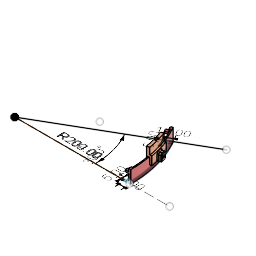
telescope complet (Autodesk Fusion 360 archive; units mm, degrees)
design "curseur_3"
Autodesk Fusion 360 part; units mm, degrees
(part 1 of 2)
sketch "Esquisse1" plane through (0, 0, 0) normal (0, 0, 1) x (1, 0, 0) in component "plateau bas"
  arc A0 (200, 0) -> (141.4214, 141.4214) centre (0, 0) ccw
  line L0 (0, 0) -> (200, 0) construction
  line L1 (0, 0) -> (141.4214, 141.4214) construction
  line L2 (0, 0) -> (141.4214, 141.4214)
  line L3 (0, 0) -> (200, 0)
  dimension "d1" = 200
  dimension "d2" = 45
  constraint coincident A0.centre L0.start
  measures "d1" radius of A0
  measures "d2" angle of L0 L1
extrude "Extrusion1" add sketch "Esquisse1" along normal blind 19 makes body 1 in component "plateau bas"
sketch "Esquisse1 (2)" plane through (0, 0, 0) normal (0, 0, 1) x (1, 0, 0) in component "plateau haut"
  line L0 (0, 0) -> (200, 0)
  arc A0 (200, 0) -> (141.4214, 141.4214) centre (0, 0) ccw
  line L1 (0, 0) -> (141.4214, 141.4214)
  point P0 (141.4214, 141.4214)
  constraint coincident L0.start A0.centre
  constraint horizontal L0
  constraint coincident P0 A0.end
extrude "Extrusion2" add sketch "Esquisse1 (2)" along normal blind 9 separate body makes body 2 in component "plateau haut"
sketch "Esquisse1 (3)" plane through (0, 0, 0) normal (0, 0, 1) x (1, 0, 0) in component "guide"
  line L0 (0, 0) -> (200, 0) construction
  line L1 (204, 0) -> (194, 0)
  line L2 (194, 5) -> (203.9387, 5)
  line L3 (194, 5) -> (194, 0)
  line L4 (0, 0) -> (235.9451, 136.223)
  line L5 (0, 0) -> (272.446, 0) construction
  arc A0 (200, 0) -> (173.2051, 100) centre (0, 0) ccw
  arc A1 (202, 0) -> (174.9371, 101) centre (0, 0) ccw
  arc A2 (204, 0) -> (176.6692, 102) centre (0, 0) ccw
  line L6 (176.6692, 102) -> (168.0089, 97)
  line L7 (168.0089, 97) -> (170.5089, 92.6699)
  line L8 (170.5089, 92.6699) -> (179.1161, 97.6392)
  arc A3 (187.7863, 74.4331) -> (187.1312, 81.2275) centre (81.8319, 67.6458) ccw
  dimension "d1_1" = 200
  dimension "d3_1" = 202
  dimension "d4_1" = 204
  dimension "d7" = 10
  dimension "d8" = 5
  dimension "d20" = 30
  dimension "d22" = 10
  dimension "d23" = 5
  constraint coincident L0.start L4.start
  constraint coincident L0 L1.end
  constraint parallel L0 L1
  constraint coincident L2.end A2
  constraint parallel L0 L2
  constraint perpendicular L0 L3
  constraint horizontal L5
  constraint coincident L4 A0.end
  constraint coincident L4 A1.end
  constraint coincident L4 A2.end
  constraint coincident L4 L6.end
  constraint perpendicular L6 L7
  constraint coincident A2 L8.end
  constraint perpendicular L7 L8
  constraint coincident A2 A3.end
  constraint coincident A1 A3.start
  measures "d1_1" radius of A0
  measures "d3_1" radius of A1
  measures "d4_1" radius of A2
  measures "d7" distance of L1.start L1.end
  measures "d8" distance of L1.end L2.start
  measures "d20" angle of L4 L5
  measures "d22" distance of A2.end L6.end
  measures "d23" distance of L6.end L7.end
extrude "Extrusion1'" add sketch "Esquisse1 (3)" along normal blind 10 separate body contours L1 L2 A0 A1 | L2 A0 A1 L8 | L4 A0 A1 L6 L8 makes body 3 in component "guide"
extrude "Extrusion2'" add sketch "Esquisse1 (3)" along normal blind 22 contours L1 L2 A1 A2 | L1 L2 A0 A1 | L2 A1 A2 A3 | A1 A2 L8 A3 | L4 A1 A2 L6 L8 | L4 A0 A1 L6 L8 bodies 3 in component "guide"
extrude "Extrusion3" add sketch "Esquisse1 (3)" along normal blind 17 and the other way blind -14 contours L1 L2 A0 A1 | L1 L2 L3 A0 | L4 A0 L6 L7 L8 | L4 A0 A1 L6 L8 bodies 3 in component "guide"
sketch "Esquisse1 (4)" plane through (0, 0, 0) normal (0, 0, 1) x (1, 0, 0) in component "curseur"
  line L0 (0, 0) -> (183.0742, 85.3689)
  arc A0 (183.0742, 85.3689) -> (165.4687, 115.8624) centre (0, 0) ccw
  line L1 (0, 0) -> (165.4687, 115.8624)
  arc A1 (181.2616, 84.5237) -> (163.8304, 114.7153) centre (0, 0) ccw
  line L2 (0, 0) -> (188.8449, 109.0297) construction
  line L3 (165.4687, 115.8624) -> (170.3836, 119.3039)
  line L4 (183.0742, 85.3689) -> (188.512, 87.9046)
  arc A2 (188.512, 87.9046) -> (170.3836, 119.3039) centre (0, 0) ccw
  line L5 (20, 0) -> (2.5, 0)
  arc A3 (185.7025, 86.5945) -> (167.8443, 117.5258) centre (0, 0) ccw
  line L6 (177.5812, 108.3001) -> (182.7774, 111.3001)
  line L7 (182.7774, 111.3001) -> (187.7774, 102.6398)
  line L8 (187.7774, 102.6398) -> (182.5812, 99.6398)
  line L9 (173.2051, 100) -> (178.7453, 100.1704)
  line L10 (173.2051, 100) -> (176.1228, 104.7128)
  dimension "d24_1" = 10
  dimension "d33" = 5
  dimension "d38" = 208
  dimension "d47" = 25
  dimension "d56" = 200
  dimension "d57" = 202
  dimension "d66" = 2.9
  dimension "d67" = 10
  dimension "d68" = 6
  constraint coincident L0 A1.start
  constraint coincident L1 A1.end
  constraint parallel L1 L3
  constraint parallel L0 L4
  constraint coincident L0.start A0.centre
  constraint coincident L0.start L2
  constraint coincident L0.start L1
  constraint coincident L0 A0.centre
  constraint coincident L4 A3.start
  constraint coincident L3 A3.end
  constraint coincident A2 L6.start
  constraint coincident A2 L8.end
  constraint perpendicular L7 L8
  constraint perpendicular L6 L7
  constraint perpendicular L2 L7
  constraint symmetric L2 L6 L8
  constraint midpoint A1 L9.start
  constraint coincident A3 L9.end
  constraint symmetric L2 L9.start L10.start
  constraint symmetric L2 L9.end L10.end
  measures "d24_1" angle of L0 L1
  measures "d33" angle of L0 L2
  measures "d38" radius of A2
  measures "d47" angle of L0 L5
  measures "d56" radius of A1
  measures "d57" radius of A0
  measures "d66" distance of A0 A3
  measures "d67" distance of L6.end L7.end
  measures "d68" distance of L7.end L8.end
extrude "Extrusion4" add sketch "Esquisse1 (4)" along normal blind 22 and the other way blind -10 separate body contours L0 A0 A1 L9 | A0 L1 A1 L10 | A0 L9 L10 | L3 L4 A2 A3 makes body 4 at (181.3843, 88.9029, 14) makes body 5 at (172.665, 115.9775, 18) in component "curseur"
extrude "Extrusion8" add sketch "Esquisse1 (4)" along normal blind 25 and the other way blind -22 contours L0 A0 A1 L9 | A0 L1 A1 L10 | A0 L4 A3 L9 | A0 L9 L10 | A0 L3 A3 L10 | A0 A3 L9 L10 | L3 L4 A2 A3 bodies 4 5 in component "curseur"
extrude "Extrusion5" add sketch "Esquisse1 (4)" along normal blind 37 and the other way blind -25 contours L0 A0 A1 L9 | A0 L1 A1 L10 | A0 L4 A3 L9 | A0 L9 L10 | A0 L3 A3 L10 | A0 A3 L9 L10 bodies 4 in component "curseur"
extrude "Extrusion9" add sketch "Esquisse1 (4)" along normal blind 40 and the other way blind -32 contours A0 L9 L10 | A0 A3 L9 L10 bodies 4 in component "curseur"
extrude "Extrusion10" add sketch "Esquisse1 (4)" along normal blind 22 and the other way blind -10 contours A2 L6 L7 L8 bodies 4 in component "curseur"
sketch "Esquisse2" plane through (185.2774, 106.9699, 0) normal (0.866025, 0.5, 0) x (-0.5, 0.866025, 0) in component "curseur"
  line L0 (-5, 10) -> (5, 10)
  line L1 (5, 10) -> (5, 22)
  line L2 (5, 22) -> (-5, 22)
  line L3 (-5, 22) -> (-5, 10)
  circle A0 centre (0, 16) radius 2.4
  dimension "d73" = 4.8
  measures "d73" diameter of A0
extrude "Extrusion11" cut sketch "Esquisse2" against normal blind 18 contours A0 bodies 4 in component "curseur"
fillet "Congé1" radius 2.5 2 edges at (180.1793, 109.8001, 22) (185.1793, 101.1398, 22) on bodies 4 in component "curseur"
fillet "Congé2" radius 1.5 5 edges at (182.5812, 99.6398, 14.75) (182.2292, 100.2821, 21.2678) (180.1333, 104, 22) (177.9615, 107.6741, 21.2678) (177.5812, 108.3001, 14.75) on bodies 4 in component "curseur"
fillet "Congé3" radius 1 5 edges at (187.7774, 102.6398, 14.75) (187.4113, 103.274, 21.2678) (185.2774, 106.9699, 22) (183.1435, 110.6659, 21.2678) (182.7774, 111.3001, 14.75) on bodies 4 in component "curseur"
component "plateau bas" placed x (1, 0, 0) y (0, 1, 0) z (0, 0, 1) at (0, 0, 0)
component "plateau haut" placed x (1, 0, 0) y (0, 1, 0) z (0, 0, 1) at (0, 0, 33)
component "guide" placed x (1, 0, 0) y (0, 1, 0) z (0, 0, 1) at (0, 0, 5)
component "curseur" placed x (0.965926, -0.258819, 0) y (0.258819, 0.965926, 0) z (0, 0, 1) at (0, 0, 5)
named bodies: "guide"

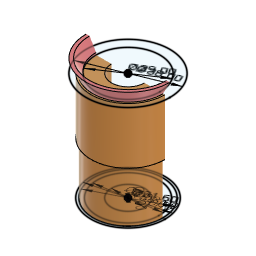
design "oculaire_20mm"
Autodesk Fusion 360 part; units mm, degrees
sketch "Esquisse1" plane through (0, 0, 0) normal (0, 0, 1) x (1, 0, 0)
  circle A0 centre (0, 0) radius 15.8
  circle A1 centre (0, 0) radius 16.8
  circle A2 centre (0, 0) radius 14
  circle A3 centre (0, 0) radius 7.5
  circle A4 centre (0, 0) radius 1
  dimension "d1" = 31.6
  dimension "d2" = 33.6
  dimension "d3" = 28
  dimension "d10" = 15
  dimension "d11" = 2
  constraint coincident A0.centre A1.centre
  constraint concentric A3 A4
  measures "d1" diameter of A0
  measures "d2" diameter of A1
  measures "d3" diameter of A2
  measures "d10" diameter of A3
  measures "d11" diameter of A4
extrude "Extrusion1" add sketch "Esquisse1" along normal blind 23.5 contours A0 makes body 1
extrude "Extrusion2" add sketch "Esquisse1" along normal blind 49 and the other way blind -23.5 contours A0 | A1 | A2 bodies 1
extrude "Extrusion4" add sketch "Esquisse1" along normal blind 40 and the other way blind -36 separate body contours A3 | A4 makes body 2
chamfer "Chanfrein1" distance 7 distance2 2 1 edges at (-6.9925, -2.7121, 40) measured on face at (1.9158, 2.8099, 40) on bodies 2
chamfer "Chanfrein2" distance 1.5 distance2 7 1 edges at (-6.9925, -2.7121, 36) measured on face at (7.4627, -0.7468, 36.6667) on bodies 2
extrude "Extrusion3" add sketch "Esquisse1" along normal blind 43 and the other way blind -23 separate body contours A4 makes body 3
sketch "Esquisse1 (2)" plane through (0, 0, 0) normal (0, 0, 1) x (1, 0, 0) in component "cahoutchouc"
  circle A0 centre (0, 0) radius 14.5
  circle A1 centre (0, 0) radius 19
  dimension "d24" = 29
  dimension "d25" = 38
  constraint coincident A0.centre A1.centre
  measures "d24" diameter of A0
  measures "d25" diameter of A1
extrude "Extrusion1'" add sketch "Esquisse1 (2)" along normal blind 6 separate body makes body 4 in component "cahoutchouc"
chamfer "Chanfrein1'" distance 3 distance2 5 1 edges at (-13.5187, 5.2434, 6) measured on face at (17.3753, -1.6643, 6) on bodies 4 in component "cahoutchouc"
chamfer "Chanfrein2'" distance 6 distance2 3 1 edges at (-17.7142, -6.8707, 0) measured on face at (18.9764, -0.9471, 4) on bodies 4 in component "cahoutchouc"
component "cahoutchouc" placed x (1, 0, 0) y (0, 1, 0) z (0, 0, 1) at (0, 0, 49)

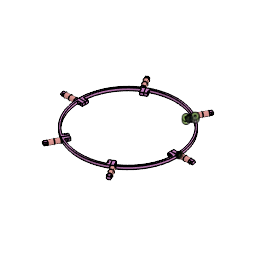
design "table a rouleau3"
Autodesk Fusion 360 part; units mm, degrees
sketch "Esquisse1" plane through (0, 0, 0) normal (0, 0, 1) x (1, 0, 0)
  line L0 (130.5, 0) -> (150, 0) construction
  arc A0 (46, 0) -> (45.9562, 2.0065) centre (0, 0) ccw
  arc A1 (47.9583, 2) -> (47.9543, 2.0937) centre (0, 0) ccw
  line L1 (130.5, 0) -> (150, 0)
  line L2 (80.1544, 120.8316) -> (72.8889, 108.2472)
  line L3 (144.7204, 9) -> (130.1893, 9)
  arc A2 (150, 0) -> (75, 129.9038) centre (0, 0) ccw
  arc A3 (144.7204, 9) -> (80.1544, 120.8316) centre (0, 0) ccw
  line L4 (186.382, -4.6913) -> (189.3792, -4.5604)
  line L5 (147.0059, 71.8492) -> (150.8185, -15.4747) construction
  line L6 (0, 0) -> (371.6459, 16.2264) construction
  line L7 (185.2639, 20.9177) -> (188.2563, 21.1586)
  line L8 (185.2639, 20.9177) -> (186.382, -4.6913)
  line L9 (188.2563, 21.1586) -> (189.3792, -4.5604)
  line L10 (65.25, 113.0163) -> (75, 129.9038)
  arc A4 (130.5, 0) -> (130.1893, 9) centre (0, 0) ccw
  arc A5 (72.8889, 108.2472) -> (65.25, 113.0163) centre (0, 0) ccw
  dimension "d2" = 150
  dimension "d6" = 46
  dimension "d7" = 48
  dimension "d13" = 145
  dimension "d49" = 2.5
  dimension "d64" = 3
  dimension "d65" = 186
  dimension "d70" = 9
  dimension "d71" = 9
  dimension "d80" = 261
  constraint horizontal L0
  constraint coincident A0.centre A1.centre
  constraint perpendicular L5 L6
  constraint tangent A2 L5
  constraint perpendicular L4 L8
  constraint perpendicular L4 L9
  constraint perpendicular L6 L8
  constraint midpoint L6 L8
  constraint coincident L6 A1.end
  constraint coincident L6 A0.end
  constraint concentric A1 A4
  constraint concentric A4 A5
  measures "d2" distance of A0.centre A2.end
  measures "d6" radius of A0
  measures "d7" radius of A1
  measures "d13" radius of A3
  measures "d49" angle of L1 L6
  measures "d64" distance of L8 L9
  measures "d65" distance of A0.centre L8
  measures "d70" distance of L2 L10
  measures "d71" distance of L1 L3
  measures "d80" diameter of A4
extrude "Extrusion1" add sketch "Esquisse1" along normal blind 8 contours L1 L2 L3 A2 A3 L10 A4 A5 makes body 1
sketch "Esquisse3" plane through (0, 0, 0) normal (-0.866025, 0.5, 0) x (-0.5, -0.866025, 0)
  line L0 (-144.5026, 0) -> (-129.5026, 0)
  line L1 (-129.5026, 0) -> (-129.5026, 8)
  line L2 (-129.5026, 8) -> (-144.5026, 8)
  line L3 (-144.5026, 8) -> (-144.5026, 0)
  circle A0 centre (-137.0026, 4) radius 2.2
  line L4 (-133.2026, 6.1939) -> (-137.0026, 8.3879)
  line L5 (-137.0026, 8.3879) -> (-140.8026, 6.1939)
  line L6 (-140.8026, 6.1939) -> (-140.8026, 1.8061)
  line L7 (-140.8026, 1.8061) -> (-137.0026, -0.3879)
  line L8 (-137.0026, -0.3879) -> (-133.2026, 1.8061)
  line L9 (-133.2026, 1.8061) -> (-133.2026, 6.1939)
  line L10 (-129.5026, 0) -> (-150, 0)
  line L11 (-150, 8) -> (-129.5026, 8)
  line L12 (-150, 0) -> (-150, 8)
  line L13 (-150, 0) -> (-130.5, 0)
  line L14 (-130.5, 8) -> (-150, 8)
  line L15 (-150, 8) -> (-150, 0)
  line L16 (-130.5, 0) -> (-130.5, 8)
  point P0 (-137.0026, 4)
  dimension "d32" = 4.4
  dimension "d33" = 7.5
  dimension "d34" = 4
  dimension "d35" = 3.8
  constraint coincident P0 A0.centre
  measures "d32" diameter of A0
  measures "d33" distance of L1 P0
  measures "d34" distance of L0 P0
  measures "d35" distance of P0 L9
extrude "Extrusion4" cut sketch "Esquisse3" along normal mid plane 30 contours A0 bodies 1
extrude "Extrusion5" cut sketch "Esquisse3" along normal blind -7 and the other way blind 15 contours L0 L2 L4 L5 L6 L7 L8 L9 L10 L11 L13 L14 bodies 1
pattern_circular "Réseau C1" count 2 over 60 about axis through (0, 0, 8) along (0, 0, -1) of "Extrusion4"
ref_plane "Plan de construction2" through (148.9122, 28.1873, 0) normal (0.999048, 0.043619, 0) x (0.043619, -0.999048, 0)
sketch "Esquisse2" plane through (149.8572, 6.5429, 0) normal (0.999048, 0.043619, 0) x (-0.043619, 0.999048, 0)
  line L0 (0, 0) -> (6, 0)
  line L1 (6, 0) -> (6, 8)
  line L2 (6, 8) -> (0, 8)
  line L3 (0, 8) -> (0, 0)
  circle A0 centre (0, 4) radius 5.5
  circle A1 centre (0, 4) radius 6.5
  line L4 (-5.1235, 0) -> (5.1235, 0)
  line L5 (-5.1235, 8) -> (5.1235, 8)
  dimension "d25" = 11
  dimension "d26" = 13
  dimension "d27" = 4
  constraint midpoint L3 A0.centre
  constraint concentric A0 A1
  constraint coincident A1 L4.start
  constraint coincident A1 L4.end
  constraint coincident L0 L4.end
  constraint parallel L0 L4
  constraint coincident A1 L5.start
  constraint coincident A1 L5.end
  constraint parallel L2 L5
  measures "d25" diameter of A0
  measures "d26" diameter of A1
  measures "d27" distance of A0.centre L5
extrude "Extrusion2" add sketch "Esquisse2" along normal blind 42 contours L0 L2 L3 A0 L4 L5 | L3 A0 L4 L5 bodies 1
extrude "Extrusion3" add sketch "Esquisse2" along normal blind 3 contours L0 L1 L2 A0 A1 L4 L5 | A0 A1 L4 L5 | L1 A1 bodies 1
extrude "Extrusion7" cut sketch "Esquisse1" along normal blind 5.5 and the other way blind -2.5 contours L4 L7 L8 L9 bodies 1
sketch "Esquisse1 (2)" plane through (0, 0, 0) normal (0, 0, 1) x (1, 0, 0) in component "rouleau"
  circle A0 centre (0, 0) radius 6
  circle A1 centre (0, 0) radius 7
  dimension "d55" = 12
  dimension "d56" = 14
  constraint coincident A0.centre A1.centre
  constraint concentric A0 A1
  measures "d55" diameter of A0
  measures "d56" diameter of A1
extrude "Extrusion1'" add sketch "Esquisse1 (2)" along normal blind 30 separate body makes body 2 in component "rouleau"
extrude "Extrusion2'" cut 1 faces at (6.6406, -0.3478, 0) along direction (0, 0, -1) blind -15.2 and the other way blind 14.8 on bodies 2 bodies 2 makes body 3 at (6.9652, -0.697, 25.0667) in component "rouleau"
pattern_circular "Réseau C2" count 6 over 360 about axis through (0, 0, 0) along (0, 0, 1) of bodies 1 makes body 4 at (56.2488, 139.0542, 5.3333) makes body 5 at (-92.3001, 118.24, 5.3333) makes body 6 at (-149.3736, -13.6942, 2.6667) makes body 7 at (-62.8273, -136.2084, 2.6667) makes body 8 at (92.3001, -118.24, 5.3333)
component_pattern "component pattern"
component "rouleau" placed x (0, 0, -1) y (0.043619, -0.999048, 0) z (-0.999048, -0.043619, 0) at (182.8258, 7.9823, 4)
component "rouleau" placed x (0, 0, -1) y (0.887011, -0.461749, 0) z (-0.461749, -0.887011, 0) at (84.5, 162.323, 4)
component "rouleau" placed x (0, 0, -1) y (0.843391, 0.5373, 0) z (0.5373, -0.843391, 0) at (-98.3258, 154.3406, 4)
component "rouleau" placed x (0, 0, -1) y (-0.043619, 0.999048, 0) z (0.999048, 0.043619, 0) at (-182.8258, -7.9823, 4)
component "rouleau" placed x (0, 0, -1) y (-0.887011, 0.461749, 0) z (0.461749, 0.887011, 0) at (-84.5, -162.323, 4)
component "rouleau" placed x (0, 0, -1) y (-0.843391, -0.5373, 0) z (-0.5373, 0.843391, 0) at (98.3258, -154.3406, 4)

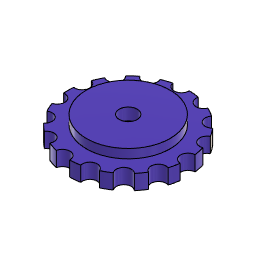
design "molette_ecrou_6"
Autodesk Fusion 360 part; units mm, degrees
sketch "Esquisse2" plane through (0, 0, 0) normal (0, 0, 1) x (1, 0, 0)
  circle A0 centre (0, 0) radius 14
  circle A1 centre (0, 0) radius 20
  circle A2 centre (20, 0) radius 2.5
  line L0 (0.202, 5.77) -> (-4.8959, 3.06)
  line L1 (-4.8959, 3.06) -> (-5.098, -2.71)
  line L2 (-5.098, -2.71) -> (-0.202, -5.77)
  line L3 (-0.202, -5.77) -> (4.8959, -3.06)
  line L4 (4.8959, -3.06) -> (5.098, 2.71)
  line L5 (5.098, 2.71) -> (0.202, 5.77)
  circle A3 centre (0, 0) radius 3
  dimension "d51_1" = 40
  dimension "d52_1" = 28
  dimension "d53_1" = 5
  dimension "d2_2" = 5
  dimension "d7_2" = 6
  constraint coincident A0.centre A1.centre
  measures "d51_1" diameter of A1
  measures "d52_1" diameter of A0
  measures "d53_1" diameter of A2
  measures "d2_2" distance of A0.centre L5
  measures "d7_2" diameter of A3
extrude "Extrusion1" add sketch "Esquisse2" along normal blind 5 contours A0 | A1 A2 | A1 A2 | L0 L1 L2 L3 L4 L5 picked at (19.214, -0.5707) picked at (17.0514, 3.8379)
extrude "Extrusion2" add sketch "Esquisse2" along normal blind 8 contours A0 | L0 L1 L2 L3 L4 L5
extrude "Extrusion3" cut sketch "Esquisse2" along normal blind 4 contours L0 L1 L2 L3 L4 L5
extrude "Extrusion6" cut sketch "Esquisse2" along normal blind 5 contours A1 A2 picked at (19.214, -0.5707)
pattern_circular "Réseau C1" count 15 over 360 about axis through (0, 0, 0) along (0, 0, 1) of "Extrusion6"

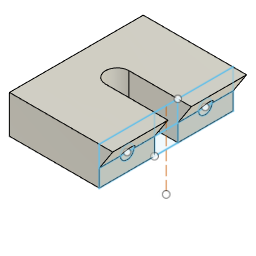
design "cale"
Autodesk Fusion 360 part; units mm, degrees
sketch "Esquisse1" plane through (-35, -25, 52.8) normal (-1, 0, 0) x (0, -1, 0)
  line L0 (14.952, -3.6934) -> (-14.848, -3.6934)
  line L1 (0.052, -3.6934) -> (0.052, -20.8144) construction
  circle A0 centre (8.7476, -8.3) radius 1.5
  circle A1 centre (-8.6437, -8.3) radius 1.5
  line L2 (-14.848, -12.1415) -> (14.952, -12.1415)
  line L3 (2.652, -3.6934) -> (2.652, -12.1415)
  line L4 (-2.548, -3.6934) -> (-2.548, -12.1415)
  line L5 (14.952, -8.3) -> (-14.848, -8.3)
  line L6 (14.952, -3.6934) -> (14.952, -12.1415)
  line L7 (-14.848, -3.6934) -> (-14.848, -12.1415)
  dimension "d166" = 3
  dimension "d167" = 2.6
  dimension "d194" = 14.9
  constraint vertical L1
  constraint symmetric L1 A0 A1
  constraint coincident L0 L3.start
  constraint perpendicular L0 L3
  constraint symmetric L1 L3.start L4.start
  constraint symmetric L1 L3.end L4.end
  constraint coincident L2 L4.end
  constraint perpendicular L2 L4
  constraint perpendicular L2 L6
  constraint symmetric L1 L0.start L0.end
  constraint symmetric L1 L2.end L2.start
  constraint coincident L0 L1.start
  constraint coincident L7 L5.end
  constraint coincident L6 L5.start
  measures "d166" diameter of A0
  measures "d167" distance of L1 L3
  measures "d194" distance of L1 L6
extrude "Extrusion1" add sketch "Esquisse1" along normal blind 20 and the other way blind 3 contours L0 A0 L3 L5 L6 | L0 L3 L4 L5 | L0 A1 L4 L5 L7
extrude "Extrusion3" add sketch "Esquisse1" along normal blind 20 contours A0 L2 L3 L5 L6 | L2 L3 L4 L5 | A1 L2 L4 L5 L7
chamfer "Chanfrein1" distance 4.6 distance2 3 3 edges at (-32, -37.5998, 44.5) (-32, -25.052, 44.5) (-32, -12.5041, 44.5) measured on face at (-32, -22.2647, 48.0585) measured on face at (-32, -22.2647, 48.0585) measured on face at (-32, -22.2647, 48.0585)
extrude "Extrusion4" cut sketch "Esquisse1" along normal blind 13.5 and the other way blind 3 contours L0 L3 L4 L5 | L2 L3 L4 L5
fillet "Congé1" radius 2.6 2 edges at (-48.5, -22.452, 44.8825) (-48.5, -27.652, 44.8825)

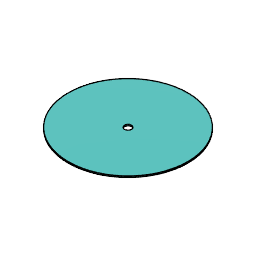
design "plaque"
Autodesk Fusion 360 part; units mm, degrees
sketch "Esquisse1" plane through (0, 0, 0) normal (0, 0, 1) x (1, 0, 0)
  circle A0 centre (0, 0) radius 70
  circle A1 centre (0, 0) radius 4.1
  dimension "d1" = 140
  dimension "d2" = 8.2
  constraint coincident A0.centre A1.centre
  constraint concentric A0 A1
  measures "d1" diameter of A0
  measures "d2" diameter of A1
extrude "Extrusion1" add sketch "Esquisse1" along normal blind 1.5
equation "d5 = 8bf455b0-8dd7-4d48-b475-9f234ed07525"

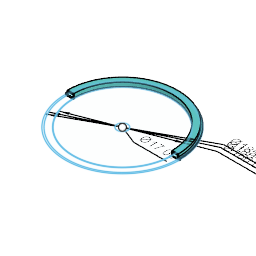
design "roulement3ext"
Autodesk Fusion 360 part; units mm, degrees
sketch "Esquisse3" plane through (0, 0, 0) normal (0, 0, 1) x (1, 0, 0)
  circle A0 centre (0, 0) radius 80
  circle A1 centre (0, 0) radius 90
  circle A2 centre (0, 0) radius 92.5
  circle A3 centre (0, 0) radius 8.5
  circle A4 centre (0, 0) radius 79.9
  dimension "d28" = 160
  dimension "d29" = 180
  dimension "d30" = 185
  dimension "d33" = 17
  constraint concentric A0 A1
  constraint concentric A1 A2
  measures "d28" diameter of A0
  measures "d29" diameter of A1
  measures "d30" diameter of A2
  measures "d33" diameter of A3
extrude "Extrusion1" add sketch "Esquisse3" along normal blind 2.5 and the other way blind -0.5 contours A1 | A2
extrude "Extrusion2" add sketch "Esquisse3" along normal blind 7 and the other way blind -0.5 contours A1
named bodies: "Corps1"

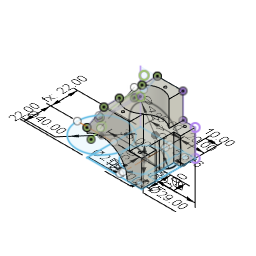
design "Bati"
Autodesk Fusion 360 part; units mm, degrees
sketch "Esquisse1" plane through (0, 0, 23) normal (0, 0, 1) x (-1, 0, 0)
  line L0 (-10, 3) -> (-10, 47)
  line L1 (-10, 47) -> (35, 47)
  line L2 (65, 25) -> (35, 25) construction
  circle A0 centre (10, 25) radius 14.5
  line L3 (10, 3.7685) -> (10, 45.0557) construction
  circle A1 centre (10, 42.5) radius 1
  line L4 (35, 3) -> (-10, 3)
  circle A2 centre (10, 7.5) radius 1
  circle A3 centre (45, 25) radius 20
  line L5 (35, 47) -> (35, 3)
  line L6 (0, 47) -> (0, 3)
  circle A4 centre (-5, 43.5) radius 1
  circle A5 centre (-5, 6.5) radius 1
  line L7 (-10, 15) -> (-4.3838, 15)
  line L8 (-4.3838, 15) -> (-4.3838, 35)
  line L9 (-4.3838, 35) -> (-10, 35)
  dimension "d71" = 29
  dimension "d72" = 20
  dimension "d75" = 17.5
  dimension "d85" = 40
  dimension "d93" = 35
  dimension "d94" = 22
  dimension "d95" = 22
  dimension "d96" = 25
  dimension "d115" = 10
  dimension "d120" = 2
  dimension "d121" = 2
  dimension "d140" = 18.5
  dimension "d141" = 5.6162
  dimension "d142" = 10
  constraint horizontal L1
  constraint coincident L2 A0.centre
  constraint coincident A0.centre L3
  constraint perpendicular L0 L4
  constraint symmetric L2 A1 A2
  constraint coincident L2 A3.centre
  constraint perpendicular L4 L5
  constraint coincident L1 L6.start
  constraint coincident L4 L6.end
  constraint perpendicular L4 L6
  constraint symmetric L2 A4 A5
  constraint coincident L0 L7.start
  constraint perpendicular L0 L7
  constraint perpendicular L7 L8
  constraint coincident L0 L9.end
  constraint perpendicular L0 L9
  constraint symmetric L2 L7 L9
  measures "d71" diameter of A0
  measures "d72" distance of L0 A0.centre
  measures "d75" distance of L2 A1.centre
  measures "d85" diameter of A3
  measures "d93" distance of A0.centre A3.centre
  measures "d94" distance of L1 L2
  measures "d95" distance of L2 L4
  measures "d96" distance of L3 L5
  measures "d115" distance of L0 L6
  measures "d120" diameter of A4
  measures "d121" diameter of A1
  measures "d140" distance of L2 A4.centre
  measures "d141" distance of L7.start L7.end
  measures "d142" distance of L2 L9
extrude "Extrusion1" add sketch "Esquisse1" along normal blind 43 contours L0 A0 L4 L6 L7 L8 | L1 A0 L4 A3 L5 L6 | L0 L1 A0 L6 L8 L9 | A0 L6 | A0 L6 L8 | A0 L8 | A3 L5 picked at (30.9179, 24.5677)
extrude "Extrusion4" cut sketch "Esquisse1" along normal blind 55 and the other way blind -26 contours A3 L5 picked at (30.9179, 24.5677)
extrude "Extrusion7" cut sketch "Esquisse1" along normal blind 50 and the other way blind -22 contours L0 A0 L4 L6 L7 L8 | L0 A0 L7 L8 L9 | L0 L1 A0 L6 L8 L9 | A0 L6 | A0 L6 L8 | A0 L8 | A4 | A5
sketch "Esquisse2" plane through (0, -3, 0) normal (0, 1, 0) x (-1, 0, 0)
  line L0 (35, 66) -> (0, 66)
  line L1 (-10, 23) -> (35, 23)
  circle A0 centre (23, 23) radius 21.35
  line L2 (-10, 23) -> (-10, 45)
  line L3 (35, 23) -> (35, 66)
  line L4 (21.0907, 66) -> (35, 44.5)
  line L5 (0, 66) -> (0, 45)
  line L6 (0, 45) -> (-10, 45)
  line L7 (-10, 45) -> (-10, 23)
  dimension "d104" = 42.7
  dimension "d105" = 33
  constraint coincident L1 A0.centre
  constraint coincident L0 L4.start
  constraint midpoint L3 L4.end
  measures "d104" diameter of A0
  measures "d105" distance of A0.centre L2
extrude "Extrusion5" cut sketch "Esquisse2" against normal blind 55 draft -0.45 contours L1 A0 L3 | L1 A0 L3
extrude "Extrusion8" cut sketch "Esquisse2" against normal blind 50 contours L0 L3 L4
sketch "Esquisse3" plane through (-44.9682, 0, 29.0918) normal (-0.839615, 0, 0.543183) x (0, -1, 0)
  line L0 (47, 18.3515) -> (47, 43.9584)
  line L1 (47, 43.9584) -> (34.3405, 43.9584)
  line L2 (15.6595, 43.9584) -> (3, 43.9584)
  line L3 (3, 43.9584) -> (3, 18.3515)
  line L4 (3, 18.3515) -> (47, 18.3515)
  ellipse E0 centre (25, -0.0586) end of major axis (25, -35.0376) minor radius 19 (38.9391, 23.7111) -> (11.0609, 23.7111) ccw
  line L5 (25, 49.3303) -> (25, -2) construction
  circle A0 centre (43.5, 30) radius 1.5
  circle A1 centre (6.5, 30) radius 1.5
  ellipse E1 centre (25, 64.3765) end of major axis (25, 37.682) minor radius 14.5 (15.6595, 43.9584) -> (34.3405, 43.9584) ccw
  line L6 (38.9391, 23.7111) -> (11.0609, 23.7111)
  line L7 (25, -15.9957) -> (25, 0.2997)
  line L8 (47, 18.3515) -> (47, 43.9584)
  line L9 (47, 43.9584) -> (34.3405, 43.9584)
  ellipse E2 centre (25, 64.3765) end of major axis (25, 37.682) minor radius 14.5 (15.6595, 43.9584) -> (34.3405, 43.9584) ccw
  line L10 (15.6595, 43.9584) -> (3, 43.9584)
  line L11 (3, 43.9584) -> (3, 18.3515)
  line L12 (3, 18.3515) -> (47, 18.3515)
  ellipse E3 centre (25, -0.0586) end of major axis (25, -36.8786) minor radius 20 (40.2742, 23.7111) -> (9.7258, 23.7111) ccw
  line L13 (40.2742, 23.7111) -> (9.7258, 23.7111)
  dimension "d112" = 3
  dimension "d139" = 18.5
  constraint perpendicular L4 L5
  constraint symmetric L5 A0 A1
  constraint coincident L5 L7.start
  measures "d112" diameter of A0
  measures "d139" distance of L5 A0.centre
extrude "Extrusion6" cut sketch "Esquisse3" against normal blind 12 contours A0 | A1
equation "d95 = d94"

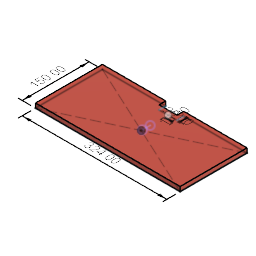
design "plaque avant"
Autodesk Fusion 360 part; units mm, degrees
sketch "Esquisse1" plane through (0, 0, 0) normal (0, 0, 1) x (1, 0, 0)
  line L0 (-162, 75) -> (-162, -75)
  line L1 (-162, -75) -> (162, -75)
  line L2 (162, -75) -> (162, 75)
  line L3 (162, 75) -> (-162, -75) construction
  line L4 (-162, 75) -> (162, -75) construction
  line L5 (20, 75) -> (20, 60)
  line L6 (20, 60) -> (0, 60)
  line L7 (0, 2.5) -> (0, 20)
  line L8 (-20, 75) -> (-20, 60)
  line L9 (-20, 60) -> (0, 60)
  line L10 (162, 75) -> (20, 75)
  line L11 (-20, 75) -> (-162, 75)
  dimension "d1" = 324
  dimension "d2" = 150
  dimension "d5" = 15
  dimension "d6" = 20
  constraint horizontal L10
  constraint perpendicular L0 L10
  constraint parallel L1 L10
  constraint parallel L0 L2
  constraint coincident L3 origin
  constraint coincident L4 origin
  constraint perpendicular L5 L10
  constraint perpendicular L5 L6
  constraint symmetric L5.start L7 L8.start
  constraint symmetric L5.end L7 L8.end
  constraint symmetric L6.end L7 L9.end
  constraint collinear L10 L11
  measures "d1" distance of L0.end L1.end
  measures "d2" distance of L0.start L0.end
  measures "d5" distance of L5.start L5.end
  measures "d6" distance of L5.end L6.end
extrude "Extrusion1" add sketch "Esquisse1" along normal blind 10

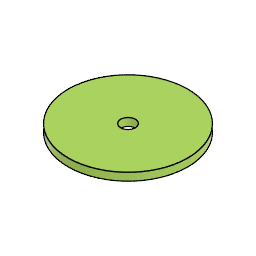
design "plaque de serrage"
Autodesk Fusion 360 part; units mm, degrees
sketch "Esquisse1" plane through (0, 0, 0) normal (0, 0, 1) x (1, 0, 0)
  circle A0 centre (0, 0) radius 69
  circle A1 centre (0, 0) radius 8.5
  dimension "d1" = 138
  dimension "d2" = 17
  constraint coincident A0.centre A1.centre
  constraint concentric A0 A1
  measures "d1" diameter of A0
  measures "d2" diameter of A1
extrude "Extrusion1" add sketch "Esquisse1" along normal blind 9

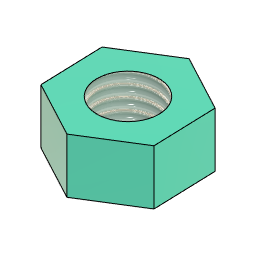
design "ecrou"
Autodesk Fusion 360 part; units mm, degrees
sketch "Esquisse1" plane through (0, 0, 0) normal (0, 0, 1) x (1, 0, 0)
  circle A0 centre (0, 0) radius 4
  line L0 (-0.2292, 6.9244) -> (-6.1113, 3.2637)
  line L1 (-6.1113, 3.2637) -> (-5.8821, -3.6607)
  line L2 (-5.8821, -3.6607) -> (0.2292, -6.9244)
  line L3 (0.2292, -6.9244) -> (6.1113, -3.2637)
  line L4 (6.1113, -3.2637) -> (5.8821, 3.6607)
  line L5 (5.8821, 3.6607) -> (-0.2292, 6.9244)
  dimension "d1" = 8
  dimension "d2" = 6
  constraint coincident A0.centre origin
  measures "d1" diameter of A0
  measures "d2" distance of A0.centre L5
extrude "Extrusion1" add sketch "Esquisse1" along normal blind 6
thread "Filetage1" "ISO Metric profile 8.0 M8x1.25 6H" major diameter 8.17 minor diameter 6.7795 pitch 1.25 angle 60 resizes the face on face at (3.995, -0.1994, 4)

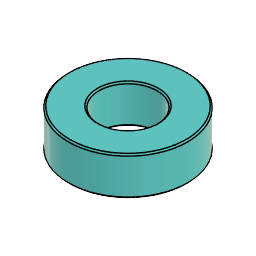
design "interieur_grand_pignon"
Autodesk Fusion 360 part; units mm, degrees
sketch "Esquisse1" plane through (0, 0, 0) normal (0, 0, 1) x (1, 0, 0)
  circle A0 centre (0, 0) radius 11
  circle A1 centre (0, 0) radius 4.1
  circle A2 centre (0, 0) radius 8.4
  dimension "d1" = 22
  dimension "d2" = 8.2
  dimension "d5" = 16.8
  constraint coincident A0.centre A1.centre
  constraint concentric A0 A1
  constraint concentric A1 A2
  measures "d1" diameter of A0
  measures "d2" diameter of A1
  measures "d5" diameter of A2
extrude "Extrusion1" add sketch "Esquisse1" along normal blind 5.4 contours A2
chamfer "Chanfrein1" distance 0.2 angle 45 4 edges at (-3.8225, 1.4826, 5.4) (-3.8225, 1.4826, 0) (-7.8315, -3.0376, 5.4) (-7.8315, -3.0376, 0)

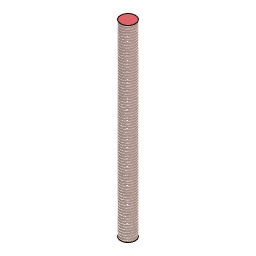
design "tige"
Autodesk Fusion 360 part; units mm, degrees
sketch "Esquisse1" plane through (0, 0, 0) normal (0, 0, 1) x (0, -1, 0)
  circle A0 centre (0, 0) radius 4
  dimension "d44" = 8
  constraint coincident A0.centre origin
  measures "d44" diameter of A0
extrude "Extrusion1" add sketch "Esquisse1" along normal blind 100
thread "Filetage1" "ISO Metric profile 8.0 M8x1.25 6g" major diameter 7.866 minor diameter 6.4455 pitch 1.25 angle 60 resizes the face on face at (-0.3983, -3.9801, 33.3333)

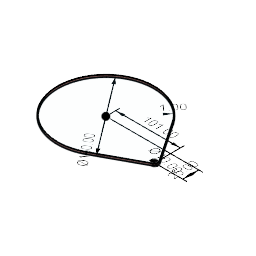
design "elastique"
Autodesk Fusion 360 part; units mm, degrees
sketch "Esquisse1" plane through (0, 0, 0) normal (0, 0, 1) x (-1, 0, 0)
  line L0 (-62.3119, -41.74) -> (-105.1541, 22.2173)
  line L1 (-103.3764, 29.3991) -> (-35.6467, 65.9872)
  arc A0 (-62.3119, -41.74) -> (-35.6467, 65.9872) centre (0, 0) ccw
  arc A1 (-103.3764, 29.3991) -> (-105.1541, 22.2173) centre (-101, 25) ccw
  line L2 (-103.8516, 30.279) -> (-36.1222, 66.867)
  arc A2 (-63.1428, -42.2964) -> (-36.1222, 66.867) centre (0, 0) ccw
  line L3 (-63.1428, -42.2964) -> (-105.985, 21.6609)
  arc A3 (-103.8516, 30.279) -> (-105.985, 21.6609) centre (-101, 25) ccw
  dimension "d2" = 10
  dimension "d3" = 150
  dimension "d4" = 101
  dimension "d5" = 25
  dimension "d6" = 1
  constraint coincident A0.centre A2.centre
  constraint tangent L0 A0
  constraint tangent L0 A1
  constraint tangent L1 A1
  constraint tangent L1 A0
  measures "d2" diameter of A1
  measures "d3" diameter of A0
  measures "d4" horizontal distance of A0.centre A1.centre
  measures "d5" vertical distance of A1.centre A0.centre
extrude "Extrusion1" add sketch "Esquisse1" along normal blind 3

design "plaque laterale gauche"
Autodesk Fusion 360 part; units mm, degrees
sketch "Esquisse1" plane through (0, 0, 0) normal (0, 0, 1) x (1, 0, 0)
  line L0 (-45, 350) -> (45, 350)
  circle A0 centre (-0.4443, 310) radius 15
  line L1 (-70, 240) -> (0, 240)
  arc A1 (25, 215) -> (0, 240) centre (0, 215) ccw
  line L2 (-95, 215) -> (-95, 65)
  line L3 (25, 215) -> (25, 65)
  line L4 (-135, 0) -> (65, 0)
  line L5 (-45, 350) -> (-135, 250)
  line L6 (0, 40) -> (-70, 40)
  arc A2 (-95, 65) -> (-70, 40) centre (-70, 65) ccw
  arc A3 (0, 40) -> (25, 65) centre (0, 65) ccw
  arc A4 (-70, 240) -> (-95, 215) centre (-70, 215) ccw
  line L7 (65, 250) -> (65, 0)
  line L8 (65, 0) -> (-135, 0)
  line L9 (-135, 250) -> (-135, 0)
  line L10 (45, 350) -> (65, 250)
  line L11 (0, 2.5) -> (0, 20)
  point P0 (5, -108)
  point P1 (-75, 200)
  dimension "d2" = 30
  dimension "d10" = 25
  dimension "d16" = 200
  dimension "d18" = 120
  dimension "d20" = 250
  dimension "d21" = 90
  dimension "d22" = 250
  dimension "d23" = 350
  dimension "d25" = 200
  dimension "d27" = 310
  dimension "d28" = 40
  dimension "d29" = 40
  dimension "d31" = 135
  dimension "d33" = 65
  dimension "d34" = 45
  dimension "d37" = 40
  dimension "d38" = 20
  dimension "d39" = 90
  constraint horizontal L0
  constraint horizontal L1
  constraint vertical L3
  constraint horizontal L6
  constraint tangent L1 A4
  constraint tangent L1 A1
  constraint equal A1 A4
  constraint tangent L3 A3
  constraint tangent L6 A3
  constraint equal A3 A4
  constraint tangent L6 A2
  constraint equal A2 A4
  constraint tangent L2 A2
  constraint tangent A1 L3
  constraint vertical L7
  constraint perpendicular L4 L9
  constraint coincident L4.end L7.end
  constraint coincident origin L4
  measures "d2" diameter of A0
  measures "d10" radius of A4
  measures "d16" distance of L1 L6
  measures "d18" distance of L2 L3
  measures "d20" distance of L4.end L7.start
  measures "d21" distance of L0.end L0.start
  measures "d22" distance of L4.start L5.end
  measures "d23" distance of L0 L4
  measures "d25" distance of L4.end L4.start
  measures "d27" distance of A0.centre L8
  measures "d28" distance of L4 L6
  measures "d29" distance of L2 L9
  measures "d31" distance of origin L9
  measures "d33" distance of origin L7
  measures "d34" distance of L0.end L11
  measures "d37" distance of A0.centre L0
  measures "d38" distance of L0.end L7
  measures "d39" distance of L0.start L9
extrude "Extrusion1" add sketch "Esquisse1" along normal blind 15

design "plateau_mobile3"
Autodesk Fusion 360 part; units mm, degrees
sketch "Esquisse1" plane through (0, 0, 0) normal (0, 0, 1) x (-1, 0, 0)
  circle A0 centre (0, 0) radius 200
  circle A1 centre (0, 0) radius 200
  line L0 (-86.4581, -25) -> (-140, -25)
  line L1 (-20, 0) -> (-2.5, 0)
  line L2 (-140, 20) -> (-140, -25)
  line L3 (0, 0) -> (177.5, 0) construction
  arc A2 (-86.4581, -25) -> (-62.5374, 64.7231) centre (0, 0) ccw
  line L4 (-20, 0) -> (-2.5, 0)
  line L5 (0, 0) -> (49.3838, 58.8533) construction
  line L6 (161.5137, -36.2069) -> (60.2712, -156.863) construction
  line L7 (-63.7034, 152.7727) -> (-164.9459, 32.1166) construction
  circle A3 centre (-114, -32) radius 2.5
  line L8 (-140, 20) -> (-62.5374, 64.7231)
  point P0 (-200, 0)
  dimension "d3" = 400
  dimension "d4" = 180
  dimension "d26" = 294
  dimension "d27" = 5
  dimension "d28" = 7
  dimension "d30" = 114
  dimension "d33" = 25
  dimension "d34" = 140
  dimension "d36" = 30
  dimension "d37" = 20
  dimension "d38" = 45
  dimension "d39" = 60
  dimension "d40" = 50
  constraint coincident A0.centre A1.centre
  constraint horizontal L0
  constraint horizontal L3
  constraint parallel L5 L6
  constraint symmetric L5 L6.start L7.start
  constraint symmetric L5 L6.end L7.end
  constraint vertical L2
  constraint coincident A0 P0
  measures "d3" diameter of A1
  measures "d4" diameter of A2
  measures "d26" distance of L6 L7
  measures "d27" diameter of A3
  measures "d28" distance of L0 A3.centre
  measures "d30" horizontal distance of A0.centre A3.centre
  measures "d33" distance of L0 L1
  measures "d34" distance of A0.centre L2
  measures "d36" angle of L1 L8
  measures "d37" distance of L1 L2.start
  measures "d38" distance of L0.end L2.start
  measures "d39" distance of L2 P0
  measures "d40" angle of L3 L5
extrude "Extrusion1" add sketch "Esquisse1" along normal blind 9
ref_plane "Plan de construction1" through (-24.6919, -29.4267, 0) normal (0.766044, -0.642788, 0) x (-0.642788, -0.766044, 0)

design "stepper"
Autodesk Fusion 360 part; units mm, degrees
sketch "Esquisse1" plane through (0, 0, 0) normal (1, 0, 0) x (0, 1, 0)
  line L0 (-28.6271, 8) -> (28.6271, 8) construction
  circle A0 centre (0, 8) radius 2.5
  circle A1 centre (0, 8) radius 4.65
  line L1 (-2, 9.5) -> (2, 9.5)
  line L2 (-2, 6.5) -> (2, 6.5)
  circle A2 centre (0, 0) radius 14
  line L3 (13.5554, 3.5) -> (17.5, 3.5)
  arc A3 (17.5, -3.5) -> (17.5, 3.5) centre (17.5, 0) ccw
  line L4 (17.5, -3.5) -> (13.5554, -3.5)
  circle A4 centre (17.5, 0) radius 1.75
  line L5 (1.75, 0) -> (22.5, 0)
  line L6 (0, 2.5) -> (0, 20)
  line L7 (-13.5554, 3.5) -> (-17.5, 3.5)
  arc A5 (-17.5, 3.5) -> (-17.5, -3.5) centre (-17.5, 0) ccw
  line L8 (-17.5, -3.5) -> (-13.5554, -3.5)
  circle A6 centre (-17.5, 0) radius 1.75
  line L9 (7, -12.0471) -> (7, -17)
  line L10 (7, -17) -> (-7, -17)
  line L11 (-7, -17) -> (-7, -12.1244)
  line L12 (7, -12.0471) -> (3.3135, -13.6022) construction
  line L13 (0, 1.75) -> (0, 22.5)
  dimension "d4_1" = 5
  dimension "d5_1" = 8
  dimension "d9" = 9.3
  dimension "d21" = 1.5
  dimension "d26" = 28
  dimension "d27" = 3.5
  dimension "d28" = 7
  dimension "d29" = 17.5
  dimension "d34" = 14
  dimension "d35" = 17
  constraint horizontal L0
  constraint midpoint L0 A0.centre
  constraint concentric A0 A1
  constraint coincident A0 L1.start
  constraint coincident A0 L1.end
  constraint horizontal L1
  constraint symmetric L0 L1.start L2.start
  constraint symmetric L0 L1.end L2.end
  constraint coincident A2.centre origin
  constraint coincident A2 L3.start
  constraint horizontal L3
  constraint tangent L3 A3
  constraint coincident A2 L4.end
  constraint parallel L3 L4
  constraint concentric A3 A4
  constraint symmetric L3 L4 L5
  constraint tangent A3 L4
  constraint symmetric L3.start L6 L7.start
  constraint symmetric L3.end L6 L7.end
  constraint symmetric A3.start L6 A5.end
  constraint symmetric A3 L6 A5
  constraint symmetric L4.end L6 L8.end
  constraint symmetric A4 L6 A6
  constraint parallel L9 L11
  constraint coincident A2 L11.end
  constraint coincident A2 L12.end
  constraint horizontal L10
  constraint vertical L11
  measures "d4_1" diameter of A0
  measures "d5_1" distance of A2.centre L0
  measures "d9" diameter of A1
  measures "d21" distance of L0 L1
  measures "d26" diameter of A2
  measures "d27" diameter of A4
  measures "d28" distance of L3 L4
  measures "d29" horizontal distance of A2.centre A3.centre
  measures "d34" distance of L9 L11
  measures "d35" distance of A2.centre L10
extrude "Extrusion1" add sketch "Esquisse1" along normal blind 1.5 contours A0 A1 L6 L13 | A0 A1 L6 L13
extrude "Extrusion5" add sketch "Esquisse1" along normal blind 10 contours A0 L1 L2 L6 L13 | A0 L1 L6 L13 | A0 L2 L6 L13 | A0 L1 L6 L13 | A0 L1 L2 L6 L13 | A0 L2 L6 L13
extrude "Extrusion2" cut sketch "Esquisse1" along normal blind 10 and the other way blind -4 contours A0 L1 L6 L13 | A0 L2 L6 L13 | A0 L1 L6 L13 | A0 L2 L6 L13
extrude "Extrusion6" add sketch "Esquisse1" against normal blind 19.5 contours A0 L1 L2 L6 L13 | A0 A1 L6 L13 | A0 L1 L6 L13 | A0 L2 L6 L13 | A0 L1 L6 L13 | A0 A1 L6 L13 | A0 L1 L2 L6 L13 | A0 L2 L6 L13 | A2 | A2 L9 L10 L11
extrude "Extrusion7" add sketch "Esquisse1" against normal blind 0.8 contours A2 A3 L4 A4 L5 | A2 L3 A3 A4 L5 | A2 L7 A5 L8

design "entretoise ext"
Autodesk Fusion 360 part; units mm, degrees
sketch "Esquisse1" plane through (0, 0, 0) normal (0, 0, 1) x (1, 0, 0)
  circle A0 centre (0, 0) radius 11
  circle A1 centre (0, 0) radius 4.1
  circle A2 centre (0, 0) radius 8.4
  dimension "d1" = 22
  dimension "d2" = 8.2
  dimension "d5" = 16.8
  constraint coincident A0.centre A1.centre
  constraint concentric A0 A1
  constraint concentric A1 A2
  measures "d1" diameter of A0
  measures "d2" diameter of A1
  measures "d5" diameter of A2
extrude "Extrusion1" add sketch "Esquisse1" along normal blind 5 contours A2
extrude "Extrusion2" add sketch "Esquisse1" along normal blind 2.4 contours A0

design "rondelle"
Autodesk Fusion 360 part; units mm, degrees
sketch "Esquisse1" plane through (0, 0, 0) normal (1, 0, 0) x (0, 1, 0)
  circle A0 centre (0, 0) radius 4.05
  circle A1 centre (0, 0) radius 11
  dimension "d144" = 8.1
  dimension "d145" = 22
  constraint coincident A0.centre A1.centre
  constraint concentric A0 A1
  measures "d144" diameter of A0
  measures "d145" diameter of A1
extrude "Extrusion1" add sketch "Esquisse1" along normal blind 1.5

design "vis de 8_molette"
Autodesk Fusion 360 part; units mm, degrees
sketch "Esquisse1" plane through (0, 0, 0) normal (0, 0, 1) x (1, 0, 0)
  circle A0 centre (0, 0) radius 40
  circle A1 centre (0, 0) radius 15
  line L0 (6, 3.4641) -> (0, 6.9282)
  line L1 (0, 6.9282) -> (-6, 3.4641)
  line L2 (-6, 3.4641) -> (-6, -3.4641)
  line L3 (-6, -3.4641) -> (0, -6.9282)
  line L4 (0, -6.9282) -> (6, -3.4641)
  line L5 (6, -3.4641) -> (6, 3.4641)
  circle A2 centre (40, 0) radius 5
  circle A3 centre (0, 0) radius 4.05
  dimension "d21" = 80
  dimension "d26" = 30
  dimension "d27" = 6
  dimension "d122" = 8.1
  constraint coincident A0.centre A1.centre
  constraint concentric A0 A1
  constraint coincident A0 A2.centre
  constraint concentric A1 A3
  measures "d21" diameter of A0
  measures "d26" diameter of A1
  measures "d27" distance of A0.centre L0
  measures "d122" diameter of A3
extrude "Extrusion1" add sketch "Esquisse1" along normal blind 6 contours A0 A2 picked at (28.6857, 8.6025)
extrude "Extrusion2" add sketch "Esquisse1" along normal blind 12 contours A1
extrude "Extrusion3" add sketch "Esquisse1" along normal blind 8 contours L0 L1 L2 L3 L4 L5
pattern_circular "Réseau C1" count 15 over 360 about axis through (0, 0, 0) along (0, 0, 1) of 1 faces at (39.2118, -4.9375, 4)

design "demi manchon"
Autodesk Fusion 360 part; units mm, degrees
sketch "Esquisse1" plane through (0, 0, 0) normal (0, 0, 1) x (0, -1, 0)
  circle A0 centre (0, 0) radius 4.05
  circle A1 centre (0, 0) radius 11
  circle A2 centre (0, 0) radius 8.4
  dimension "d103_1" = 8.1
  dimension "d123" = 16.8
  dimension "d8" = 22
  constraint coincident A0.centre A1.centre
  constraint concentric A1 A2
  measures "d103_1" diameter of A0
  measures "d123" diameter of A2
  measures "d8" diameter of A1
extrude "Extrusion1" add sketch "Esquisse1" along normal blind 8.4 contours A1 | A2
extrude "Extrusion2" add sketch "Esquisse1" against normal blind 3 contours A2

design "renfort"
Autodesk Fusion 360 part; units mm, degrees
sketch "Esquisse1" plane through (0, 0, 0) normal (0, 0, 1) x (1, 0, 0)
  line L0 (-45, 0) -> (45, 0)
  line L1 (45, 0) -> (45, 90)
  line L2 (45, 90) -> (-45, 90)
  line L3 (-45, 90) -> (-45, 0)
  circle A0 centre (0, 45) radius 15
  dimension "d1" = 90
  dimension "d2" = 90
  dimension "d3" = 30
  dimension "d4" = 45
  dimension "d5" = 45
  constraint horizontal L0
  constraint vertical L1
  constraint horizontal L2
  constraint vertical L3
  constraint coincident origin L0
  measures "d1" distance of L0.start L0.end
  measures "d2" distance of L0.start L2.end
  measures "d3" diameter of A0
  measures "d4" distance of L2 A0.centre
  measures "d5" distance of L1 A0.centre
extrude "Extrusion1" add sketch "Esquisse1" along normal blind 14

design "interieur_tube_carré"
Autodesk Fusion 360 part; units mm, degrees
sketch "Esquisse1" plane through (0, 0, 0) normal (0, 0, 1) x (1, 0, 0)
  circle A0 centre (0, 0) radius 4.1
  circle A1 centre (0, 0) radius 8.25
  dimension "d2" = 8.2
  dimension "d5" = 16.5
  constraint concentric A0 A1
  measures "d2" diameter of A0
  measures "d5" diameter of A1
extrude "Extrusion1" add sketch "Esquisse1" along normal blind 20
chamfer "Chanfrein1" distance 0.2 angle 45 4 edges at (-3.8225, 1.4826, 20) (-3.8225, 1.4826, 0) (-7.6917, -2.9833, 20) (-7.6917, -2.9833, 0)

design "carré"
Autodesk Fusion 360 part; units mm, degrees
sketch "Esquisse1" plane through (0, 0, 0) normal (0, 1, 0) x (-1, 0, 0)
  line L0 (10, 10) -> (-10, 10)
  line L1 (-10, 10) -> (-10, -10)
  line L2 (-10, -10) -> (10, -10)
  line L3 (10, -10) -> (10, 10)
  line L4 (10, 10) -> (-10, -10) construction
  line L5 (-10, 10) -> (10, -10) construction
  line L6 (-8.6914, -8.6914) -> (8.6914, -8.6914)
  line L7 (8.6914, -8.6914) -> (8.6914, 8.6914)
  line L8 (8.6914, 8.6914) -> (-8.6914, 8.6914)
  line L9 (-8.6914, 8.6914) -> (-8.6914, -8.6914)
  dimension "d124" = 20
  dimension "d125" = 20
  dimension "d126" = -1.3086
  constraint horizontal L0
  constraint perpendicular L0 L1
  constraint parallel L0 L2
  constraint parallel L1 L3
  constraint coincident L4 origin
  constraint coincident L5 origin
  measures "d124" distance of L1.end L2.end
  measures "d125" distance of L0.end L1.end
extrude "Extrusion1" add sketch "Esquisse1" along normal mid plane 100
sketch "Esquisse3" plane through (0, 0, 10) normal (0, 0, 1) x (-1, 0, 0)
  line L0 (-10, 50) -> (-10, -50)
  line L1 (-10, -50) -> (10, -50)
  line L2 (10, -50) -> (10, 50)
  line L3 (10, 50) -> (-10, 50)
  line L4 (-10, -50) -> (10, 50) construction
  line L5 (-10, 50) -> (10, -50) construction
  circle A0 centre (0, 0) radius 8
  dimension "d164" = 16
  constraint coincident L0.end L1.start
  constraint coincident L2.end L3.start
  constraint coincident L0.start L3.end
  constraint coincident L1.end L2.start
  constraint midpoint L4 A0.centre
  measures "d164" diameter of A0
extrude "Extrusion2" cut sketch "Esquisse3" against normal up to surface (20 mm away) contours A0
sketch "Esquisse4" plane through (10, 0, 0) normal (1, 0, 0) x (0, 1, 0)
  line L0 (-50, -10) -> (50, -10)
  line L1 (50, -10) -> (50, 10)
  line L2 (50, 10) -> (-50, 10)
  line L3 (-50, 10) -> (-50, -10)
  line L4 (0, 10) -> (0, -10) construction
  line L5 (-35, -3.1) -> (-15, -3.1)
  arc A0 (-15, -3.1) -> (-15, 3.1) centre (-15, 0) ccw
  line L6 (-15, 3.1) -> (-35, 3.1)
  arc A1 (-35, 3.1) -> (-35, -3.1) centre (-35, 0) ccw
  line L7 (-35, 0) -> (-15, 0) construction
  line L8 (0, 1.75) -> (0, 22.5)
  dimension "d213" = 6.2
  dimension "d214" = 20
  dimension "d219" = 15
  constraint midpoint L2 L4.start
  constraint midpoint L0 L4.end
  constraint tangent L5 A0
  constraint tangent A0 L6
  constraint parallel L5 L6
  constraint tangent L6 A1
  constraint tangent L5 A1
  constraint parallel L2 L7
  measures "d213" diameter of A0
  measures "d214" distance of A1.centre A0.centre
  measures "d219" distance of A0.centre L8
extrude "Extrusion3" cut sketch "Esquisse4" against normal blind 25 contours L5 A0 L6 A1
mirror "Symétrie miroir1" about plane through (0, 0, 0) normal (0, 1, 0) of "Extrusion3"

design "cale"
Autodesk Fusion 360 part; units mm, degrees
sketch "Esquisse1" plane through (0, 0, 0) normal (0, 0, 1) x (1, 0, 0)
  circle A0 centre (0.0297, -0.0179) radius 100
  circle A1 centre (0.0297, -0.0179) radius 45
  line L0 (20, 0) -> (2.5, 0) construction
  arc A2 (49.8264, -4.5217) -> (50.0296, 0.0422) centre (0.0297, -0.0179) ccw
  line L1 (51.9728, -7.2232) -> (91.5934, -12.7191)
  arc A3 (49.8264, -4.5217) -> (51.9728, -7.2232) centre (52.3163, -4.7469) ccw
  arc A4 (94.4216, -10.5193) -> (95.0039, 0.0008) centre (0.0297, -0.0179) ccw
  arc A5 (91.5934, -12.7191) -> (94.4216, -10.5193) centre (91.9369, -10.2428) ccw
  arc A6 (50.0296, -0.0422) -> (49.8264, 4.5217) centre (0.0297, 0.0179) ccw
  arc A7 (51.9728, 7.2232) -> (49.8264, 4.5217) centre (52.3163, 4.7469) ccw
  line L2 (51.9728, 7.2232) -> (91.5934, 12.7191)
  arc A8 (94.4216, 10.5193) -> (91.5934, 12.7191) centre (91.9369, 10.2428) ccw
  arc A9 (95.0039, -0.0008) -> (94.4216, 10.5193) centre (0.0297, 0.0179) ccw
  dimension "d1" = 200
  dimension "d3" = 90
  dimension "d7" = 100
  dimension "d16" = 2.5
  dimension "d17" = 2.5
  dimension "d18" = 40
  constraint concentric A0 A1
  constraint concentric A1 A2
  constraint tangent A2 A3
  constraint tangent L1 A3
  constraint coincident A0.centre A1.centre
  constraint tangent L1 A5
  constraint tangent A4 A5
  constraint symmetric L0 A2 A6
  constraint symmetric L0 A2.end A6.start
  constraint symmetric L0 L1.start A7.start
  constraint symmetric L0 A2.start A6.end
  constraint symmetric L0 A3 A7
  constraint symmetric L0 A4.end A9.start
  constraint symmetric L0 A4 A9
  constraint symmetric L0 L1.end L2.end
  constraint symmetric L0 A4.start A8.start
  constraint symmetric L0 A5 A8
  measures "d1" diameter of A0
  measures "d3" diameter of A1
  measures "d7" diameter of A2
  measures "d16" radius of A3
  measures "d17" radius of A5
  measures "d18" distance of L1.start L1.end
extrude "Extrusion1" add sketch "Esquisse1" along normal blind 5 contours A0 | A2 L1 A3 A4 A5 A6 A7 L2 A8 A9
extrude "Extrusion2" cut sketch "Esquisse1" along normal blind 10 contours A2 L1 A3 A4 A5 A6 A7 L2 A8 A9
pattern_circular "Réseau C1" count 18 over 360 about axis through (0.0297, -0.0179, 5) along (0, 0, 1) of "Extrusion2"
chamfer "Chanfrein1" [suppressed]

design "molette"
Autodesk Fusion 360 part; units mm, degrees